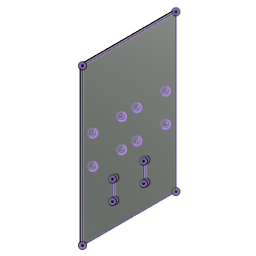
Chassis frame v6 (Autodesk Fusion 360 design; units mm, degrees)
Autodesk Fusion 360 part; units mm, degrees
sketch "Sketch1" plane through (0, 0, 0) normal (1, 0, 0) x (0, 1, 0) in component "Motor driver fitter"
  line L0 (-22.5, -22.5) -> (22.5, -22.5)
  line L1 (-47.5, -12.5) -> (-47.5, 12.5)
  line L2 (-22.5, -12.5) -> (-47.5, -12.5)
  circle A0 centre (-29, 6) radius 1.5
  circle A1 centre (-41, -6) radius 1.5
  line L3 (-47.5, 12.5) -> (-22.5, 12.5)
  line L4 (22.5, 22.5) -> (-22.5, 22.5)
  line L5 (22.5, -22.5) -> (22.5, 22.5)
  circle A2 centre (-18.5, 18.5) radius 1.5
  line L6 (-22.5, 22.5) -> (22.5, -22.5) construction
  line L7 (-22.5, -22.5) -> (22.5, 22.5) construction
  circle A3 centre (18.5, 18.5) radius 1.55
  circle A4 centre (-18.5, -18.5) radius 1.55
  circle A5 centre (18.5, -18.5) radius 1.55
  line L8 (-22.5, 22.5) -> (-22.5, 12.5)
  line L9 (-22.5, -12.5) -> (-22.5, -22.5)
  line L10 (-22.5, 12.5) -> (-47.5, -12.5) construction
  line L11 (-41, -6) -> (-47.5, -12.5) construction
  line L12 (-29, 6) -> (-22.5, 12.5) construction
  dimension "d171" = 45
  dimension "d172" = 45
  dimension "d174" = 3
  dimension "d185" = 3
  dimension "d186" = 3
  dimension "d188" = 25
  dimension "d189" = 25
  dimension "d192" = 18.5
  dimension "d193" = 18.5
  dimension "d225" = 16.9706
  constraint horizontal L0
  constraint horizontal L4
  constraint horizontal L2
  constraint vertical L1
  constraint horizontal L3
  constraint vertical L5
  constraint equal L2 L3
  constraint midpoint L6 origin
  constraint perpendicular L3 L8
  constraint perpendicular L0 L9
  constraint equal L8 L9
  constraint coincident A0.centre L10
  constraint coincident A1.centre L10
  constraint coincident A1.centre L11.start
  constraint parallel L10 L11
  constraint coincident A0.centre L12.start
  constraint parallel L10 L12
  constraint equal L11 L12
  measures "d171" distance of L0.start L0.end
  measures "d172" distance of L0.start L4.end
  measures "d174" diameter of A2
  measures "d185" diameter of A1
  measures "d186" diameter of A0
  measures "d188" distance of L1.end L1.start
  measures "d189" distance of L2.start L1.start
  measures "d192" horizontal distance of A2.centre origin
  measures "d193" vertical distance of A2.centre origin
  measures "d225" distance of A1.centre A0.centre
sketch "Sketch1 (2)" plane through (0, 0, 0) normal (1, 0, 0) x (0, 1, 0) in component "Chassis frame"
  line L0 (-125, 12.5) -> (-125, -12.5)
  circle A0 centre (-106.461, -5.961) radius 1.5
  line L1 (125, -12.5) -> (125, 12.5)
  line L2 (125, 12.5) -> (-125, 12.5)
  circle A1 centre (-118.4999, 5.9999) radius 1.5
  line L3 (-125, -12.5) -> (125, -12.5)
  line L4 (-125, 12.5) -> (125, -12.5) construction
  line L5 (-125, -12.5) -> (125, 12.5) construction
  line L6 (-22.5, 22.5) -> (22.5, -22.5)
  circle A2 centre (-6, 115) radius 1.55
  circle A3 centre (6, 103) radius 1.55
  line L7 (0, 12.5) -> (0, -12.5) construction
  line L8 (-125, 12.5) -> (-100, -12.5) construction
  line L9 (-125, 12.5) -> (-91.4846, 12.5) construction
  line L10 (-125, 12.5) -> (-118.4999, 5.9999) construction
  line L11 (-106.461, -5.961) -> (-100, -12.5) construction
  circle A4 centre (118.4999, 5.9999) radius 1.5
  circle A5 centre (106.461, -5.961) radius 1.5
  circle A6 centre (-49.7943, -5.961) radius 1.5
  circle A7 centre (-61.8332, 5.9999) radius 1.5
  circle A8 centre (6.8724, -5.961) radius 1.5
  circle A9 centre (-5.1666, 5.9999) radius 1.5
  circle A10 centre (63.539, -5.961) radius 1.5
  circle A11 centre (51.5001, 5.9999) radius 1.5
  point P0 (22, -6.0625)
  dimension "d199" = 250
  dimension "d200" = 25
  dimension "d201" = 3
  dimension "d202" = 3
  dimension "d231" = 45
  dimension "d232" = 16.9706
  dimension "d235" = 170
  dimension "d236" = 0
  constraint horizontal L2
  constraint perpendicular L0 L2
  constraint parallel L2 L3
  constraint parallel L0 L1
  constraint midpoint L4 origin
  constraint midpoint L2 L7.start
  constraint midpoint L3 L7.end
  constraint horizontal L9
  constraint coincident L3 L8.end
  constraint coincident A1.centre L8
  constraint coincident A1.centre L10.end
  constraint coincident A0.centre L11.start
  constraint equal L10 L11
  constraint symmetric A0 L7 A5
  constraint symmetric A1 L7 A4
  measures "d199" distance of L0.end L1.start
  measures "d200" distance of L0.end L0.start
  measures "d201" diameter of A0
  measures "d202" diameter of A1
  measures "d231" angle of L8 L9
  measures "d232" distance of A0.centre A1.centre
sketch "Sketch1 (3)" plane through (0, 0, 0) normal (1, 0, 0) x (0, 1, 0) in component "Motor fitter"
  line L0 (-12.5, -45) -> (-12.5, 45)
  line L1 (-12.5, 45) -> (12.5, 45)
  line L2 (12.5, 45) -> (12.5, -45)
  line L3 (12.5, -45) -> (-12.5, -45)
  line L4 (-12.5, -45) -> (12.5, 45) construction
  line L5 (-12.5, 45) -> (12.5, -45) construction
  line L6 (-12.5, 45) -> (12.5, 20) construction
  line L7 (-12.5, 45) -> (24.7988, 45) construction
  circle A0 centre (-6, 38.5) radius 1.5 construction
  circle A1 centre (6, 26.5) radius 1.5 construction
  line L8 (6, 26.5) -> (12.5, 20) construction
  line L9 (-6, 38.5) -> (-12.5, 45) construction
  dimension "d222" = 25
  dimension "d223" = 90
  dimension "d227" = 45
  dimension "d228" = 3
  dimension "d229" = 3
  dimension "d230" = 16.9706
  constraint horizontal L1
  constraint vertical L2
  constraint horizontal L3
  constraint vertical L0
  constraint midpoint origin L5
  constraint horizontal L7
  constraint coincident L2 L6.end
  constraint coincident L6 A0.centre
  constraint coincident L6 A1.centre
  constraint coincident A1.centre L8.start
  constraint coincident A0.centre L9.start
  constraint parallel L6 L9
  constraint equal L8 L9
  measures "d222" distance of L0.end L1.end
  measures "d223" distance of L2.end L1.end
  measures "d227" angle of L6 L7
  measures "d228" diameter of A0
  measures "d229" diameter of A1
  measures "d230" distance of A0.centre A1.centre
sketch "Sketch1 (4)" plane through (0, 0, 0) normal (1, 0, 0) x (0, 1, 0) in component "Breadboard fitter"
  line L0 (-65, 12.5) -> (-40, 12.5)
  line L1 (-40, 12.5) -> (-40, -12.5)
  line L2 (-40, -12.5) -> (-65, -12.5)
  line L3 (-65, -12.5) -> (-65, 12.5)
  line L4 (40, 25) -> (-40, 25)
  line L5 (-40, 25) -> (-40, -25)
  line L6 (-40, -25) -> (40, -25)
  line L7 (40, -25) -> (40, 25)
  line L8 (40, 25) -> (-40, -25) construction
  line L9 (-40, 25) -> (40, -25) construction
  circle A0 centre (-57.0753, -4.5753) radius 1.5 construction
  circle A1 centre (-47.9247, 4.5753) radius 1.5 construction
  line L10 (-47.9247, 4.5753) -> (-40, 12.5) construction
  line L11 (-57.0753, -4.5753) -> (-65, -12.5) construction
  dimension "d237" = 25
  dimension "d238" = 25
  dimension "d239" = 80
  dimension "d240" = 50
  dimension "d241" = 3
  dimension "d242" = 3
  dimension "d244" = 12.9408
  dimension "d245" = 45
  constraint horizontal L0
  constraint vertical L1
  constraint horizontal L2
  constraint vertical L3
  constraint horizontal L4
  constraint perpendicular L4 L5
  constraint parallel L4 L6
  constraint parallel L5 L7
  constraint coincident L8 origin
  constraint coincident L9 origin
  constraint midpoint L1 L5
  constraint coincident A1.centre L10.start
  constraint coincident A0.centre L11.start
  constraint equal L10 L11
  constraint parallel L10 L11
  measures "d237" distance of L0.start L0.end
  measures "d238" distance of L0.start L2.end
  measures "d239" distance of L5.end L6.end
  measures "d240" distance of L4.end L5.end
  measures "d241" diameter of A0
  measures "d242" diameter of A1
  measures "d244" distance of A0.centre A1.centre
  measures "d245" angle of L2 L11
sketch "Sketch1 (5)" plane through (0, 0, 0) normal (1, 0, 0) x (0, 1, 0) in component "Integrated frame"
  circle A0 centre (-46.8244, 18.5) radius 1.5
  circle A1 centre (-9.8244, 18.5) radius 1.5
  circle A2 centre (-46.8244, -18.5) radius 1.5
  circle A3 centre (-9.8244, -18.5) radius 1.5
  line L0 (0, 0) -> (0, 35.4619) construction
  line L1 (60, 100) -> (-60, 100)
  line L2 (-60, 100) -> (-60, -100)
  line L3 (-60, -100) -> (60, -100)
  line L4 (60, -100) -> (60, 100)
  line L5 (60, 100) -> (-60, -100) construction
  line L6 (-60, 100) -> (60, -100) construction
  circle A4 centre (46.8244, 18.5) radius 1.5
  circle A5 centre (46.8244, -18.5) radius 1.5
  circle A6 centre (9.8244, -18.5) radius 1.5
  circle A7 centre (9.8244, 18.5) radius 1.5
  line L7 (-18.5, -45.3481) -> (-21.5, -45.3481)
  line L8 (-21.5, -45.3481) -> (-21.5, -70.3481)
  line L9 (-21.5, -70.3481) -> (-18.5, -70.3481)
  line L10 (-18.5, -70.3481) -> (-18.5, -45.3481)
  line L11 (21.5, -45.3481) -> (21.5, -70.3481)
  line L12 (18.5, -70.3481) -> (18.5, -45.3481)
  line L13 (18.5, -45.3481) -> (21.5, -45.3481)
  line L14 (21.5, -70.3481) -> (18.5, -70.3481)
  point P0 (-28.3244, 0)
  dimension "d246" = 3
  dimension "d248" = 18.5
  dimension "d249" = 18.5
  dimension "d252" = 37
  dimension "d253" = -37
  dimension "d261" = 120
  dimension "d262" = 200
  dimension "d264" = 3
  dimension "d265" = 25
  dimension "d266" = 18.5
  constraint coincident L0.start origin
  constraint horizontal L1
  constraint perpendicular L1 L2
  constraint parallel L1 L3
  constraint parallel L2 L4
  constraint coincident L5 L0.start
  constraint coincident L6 L0.start
  constraint symmetric A0 L0 A4
  constraint symmetric A1 L0 A7
  constraint symmetric A2 L0 A5
  constraint symmetric A3 L0 A6
  constraint horizontal P0 L0.start
  constraint horizontal L7
  constraint vertical L8
  constraint horizontal L9
  constraint vertical L10
  constraint symmetric L0 L7.start L12.end
  constraint symmetric L0 L7.end L11.start
  constraint symmetric L0 L8.end L11.end
  constraint symmetric L0 L9.end L12.start
  measures "d246" diameter of A0
  measures "d248" horizontal distance of A0.centre P0
  measures "d249" vertical distance of A0.centre P0
  measures "d261" distance of L2.end L3.end
  measures "d262" distance of L1.end L2.end
  measures "d264" distance of L7.start L7.end
  measures "d265" distance of L7.start L9.end
  measures "d266" distance of L0.start L10
extrude "Extrude1" add sketch "Sketch1 (5)" along normal blind 3 in component "Integrated frame"
sketch "Laser cut sketch" plane through (3, 0, 0) normal (1, 0, 0) x (0, 1, 0) in component "Integrated frame"
  circle A0 centre (-9.8244, -18.5) radius 1.5
  circle A1 centre (-46.8244, -18.5) radius 1.5
  circle A2 centre (-46.8244, 18.5) radius 1.5
  circle A3 centre (-9.8244, 18.5) radius 1.5
  circle A4 centre (46.8244, 18.5) radius 1.5
  circle A5 centre (46.8244, -18.5) radius 1.5
  circle A6 centre (9.8244, -18.5) radius 1.5
  circle A7 centre (9.8244, 18.5) radius 1.5
  line L0 (-18.5, -45.3481) -> (-18.5, -70.3481)
  line L1 (-18.5, -70.3481) -> (-21.5, -70.3481)
  line L2 (-21.5, -70.3481) -> (-21.5, -45.3481)
  line L3 (-21.5, -45.3481) -> (-18.5, -45.3481)
  line L4 (21.5, -45.3481) -> (21.5, -70.3481)
  line L5 (21.5, -70.3481) -> (18.5, -70.3481)
  line L6 (18.5, -70.3481) -> (18.5, -45.3481)
  line L7 (18.5, -45.3481) -> (21.5, -45.3481)
  line L8 (60, -100) -> (60, 100)
  line L9 (60, 100) -> (-60, 100)
  line L10 (-60, 100) -> (-60, -100)
  line L11 (-60, -100) -> (60, -100)
extrude "Extrude2" [suppressed]
component "Motor driver fitter" placed x (1, 0, 0) y (0, 1, 0) z (0, 0, 1) at (0, 0, 0)
component "Chassis frame" placed x (1, 0, 0) y (0, 1, 0) z (0, 0, 1) at (0, 0, 0)
component "Motor fitter" placed x (1, 0, 0) y (0, 1, 0) z (0, 0, 1) at (0, 0, 0)
component "Breadboard fitter" placed x (1, 0, 0) y (0, 1, 0) z (0, 0, 1) at (0, 0, 0)
component "Integrated frame" placed x (1, 0, 0) y (0, 1, 0) z (0, 0, 1) at (0, 0, 0)
equation "partLength = 250 mm"
equation "partWidth = 25 mm"
equation "boltHole = 3 mm"
equation "boltFromEdgesClose = 10 mm"
equation "boltGap = 12 mm"
equation "boltFromEdgesFar = 40 mm"
equation "boltGapFromSide = ( partWidth - boltGap ) / 2"
equation "d174 = boltHole"
equation "d185 = boltHole"
equation "d186 = boltHole"
equation "d192 = ( 37 / 2 ) * 1 mm"
equation "d193 = ( 37 / 2 ) * 1 mm"
equation "d199 = partLength"
equation "d200 = partWidth"
equation "d201 = boltHole"
equation "d202 = boltHole"
equation "d222 = partWidth"
equation "d225 = boltGapDiag"
equation "boltGapDiag = boltGap * sqrt(2)"
equation "d228 = boltHole"
equation "d229 = boltHole"
equation "d230 = boltGapDiag"
equation "d232 = boltGapDiag"
equation "d241 = boltHole"
equation "d242 = boltHole"
equation "d246 = boltHole"
equation "d248 = ( 37 / 2 ) * 1 mm"
equation "d249 = ( 37 / 2 ) * 1 mm"
equation "d266 = ( 37 / 2 ) * 1 mm"
